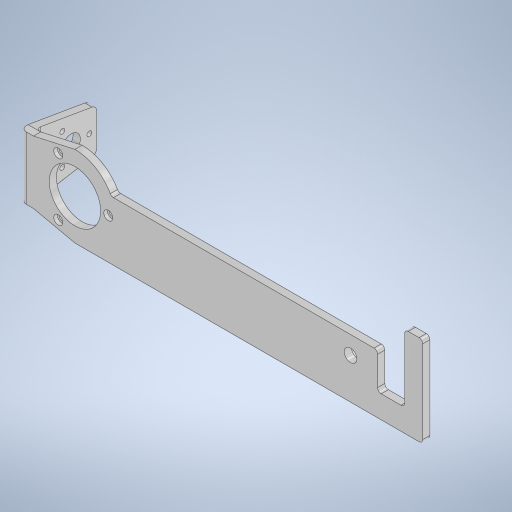
# Autodesk Inventor part: motor_holder_2
Saved by Autodesk Inventor 2024 (Build 280153000, 153)
## iProperties
Created: 2025-02-07
Part Number: motor_holder_2
Material: アルミニウム 6061
Document SubType Name: Modeling
Designer: 1412z
Density: 2.7 g/cm^3
Appearance: アルミニウム - つや出し
Author: 1412z
Autodesk Inventor part; units mm, degrees
ref_plane "YZ Plane" through (0, 0, 0) normal (1, 0, 0) x (0, 1, 0)
ref_plane "XZ Plane" through (0, 0, 0) normal (0, 1, 0) x (-1, 0, 0)
ref_plane "XY Plane" through (0, 0, 0) normal (0, 0, 1) x (1, 0, 0)
sketch "スケッチ1" plane through (0, 0, 0) normal (1, 0, 0) x (0, 1, 0)
  circle A0 centre (0, 0) radius 10
  circle A1 centre (0, -10) radius 1.35
  circle A2 centre (8.6603, 5) radius 1.35
  circle A3 centre (-8.6603, 5) radius 1.35
  circle A4 centre (0, 0) radius 5
  line L0 (0, 0) -> (0, 50)
  circle A5 centre (0, 50) radius 22.5
  circle A6 centre (0, 0) radius 14
  line L1 (-14, 0) -> (-22.5, 50)
  line L2 (14, 0) -> (22.5, 50)
  line L3 (0, -14) -> (-11.62, -14)
  line L4 (-11.62, -14) -> (-14, 0)
  line L5 (0, -14) -> (11.62, -14)
  line L6 (11.62, -14) -> (14, 0)
  line L7 (0, 20) -> (-17.4, 20)
  line L8 (0, 20) -> (17.4, 20)
  dimension "d0" = 20
  dimension "d1" = 2.7
  dimension "d4" = 360
  dimension "d6" = 10
  dimension "d7" = 50
  dimension "d8" = 45
  dimension "d9" = 28
  constraints: 18 end point, 7 point on line, 6 centre point, 6 coincident, 5 point on circle, 1 horizontal, 1 perpendicular, 1 tangent, 1 vertical, 1 vertical alignment, 10 other
  measures "d1" diameter of A1
  measures "d6" diameter of A4
  measures "d7" distance of L0.start L0.end
  measures "d8" diameter of A5
  measures "d9" diameter of A6
extrude "押し出し1" add sketch "スケッチ1" along normal blind 4 contours A0 A1 A3 A2 | A6 L6 L4 | A6 L1 L7 L0 | L0 L8 L2 A6 | L6 L5 A6 | A6 L3 L4
sketch "スケッチ2" plane through (0, -17.4, 20) normal (0, 0, 1) x (1, 0, 0)
  line L0 (0, 17.4) -> (30, 17.4)
  circle A0 centre (30, 17.4) radius 22.5
  circle A1 centre (30, 17.4) radius 18.5
  circle A2 centre (30, 17.4) radius 14.25
  circle A3 centre (48.5, 17.4) radius 1.35
  circle A4 centre (20.75, 33.4215) radius 1.35
  circle A5 centre (20.75, 1.3785) radius 1.35
  line L1 (0, 29.02) -> (0, 34.8) projected
  line L2 (0, 0) -> (0, 5.78) projected
  line L3 (0, 34.8) -> (0, 0)
  line L4 (4, 29.02) -> (4, 34.8) projected
  line L5 (4, 34.8) -> (7, 34.8)
  line L6 (7, 34.8) -> (30, 39.9)
  line L7 (4, 0) -> (4, 5.78) projected
  line L8 (4, 0) -> (7, 0)
  line L9 (7, 0) -> (30, -5.1)
  line L10 (4, 0) -> (0, 0)
  line L11 (0, 34.8) -> (4, 34.8) projected
  line L12 (0, 0) -> (0, 34.8)
  line L13 (0, 34.8) -> (4, 34.8)
  dimension "d14" = 37
  dimension "d12" = 30
  dimension "d13" = 45
  dimension "d15" = 28.5
  dimension "d16" = 2.7
  dimension "d19" = 360
  dimension "d21" = 3
  dimension "d22" = 3
  constraints: 18 end point, 5 centre point, 4 horizontal, 3 coincident, 2 point on circle, 1 collinear, 1 horizontal alignment, 1 perpendicular, 1 vertical, 9 other
  measures "d12" distance of L0.start L0.end
  measures "d13" diameter of A0
  measures "d15" diameter of A2
  measures "d16" diameter of A3
  measures "d21" distance of L4.end L5.end
  measures "d22" distance of L7.start L8.end
extrude "押し出し2" add sketch "スケッチ2" along normal blind 4 contours L3 L1 L11 L5 L6 A0 L0 | L0 A0 L9 L8 L10 L2 L3 | A1 A4 A3 A5 | A0 L6 L9
fillet "フィレット1" radius 3 2 edges at (4, 0, 20) (0, 0, 24)
fillet "フィレット2" radius 3 2 edges at (2, -11.62, -14) (2, 11.62, -14)
sketch "スケッチ7" plane through (0, -17.4, 24) normal (0, 0, 1) x (1, 0, 0)
  circle A0 centre (30, 17.4) radius 14.25 projected
  line L0 (30, 17.4) -> (182.95, 17.4)
  line L1 (30, 17.4) -> (182.95, 17.4) construction
  circle A1 centre (182.95, 17.4) radius 3.5
  circle A2 centre (182.95, 17.4) radius 10
  line L2 (182.95, 27.4) -> (50.1556, 27.4)
  arc A3 (30, -5.1) -> (30, 39.9) centre (30, 17.4) ccw projected
  line L3 (182.95, 27.4) -> (315.7444, 27.4) construction
  line L4 (182.95, 7.4) -> (50.1556, 7.4)
  point P0 (0, 17.4)
  dimension "d55" = 152.95
  dimension "d56" = 0
  dimension "d57" = 7
  dimension "d58" = 20
  dimension "d59" = 180
  constraints: 10 end point, 4 horizontal, 4 point on circle, 2 centre point, 2 coincident, 2 collinear, 1 tangent
  measures "d55" distance of L0.start L0.end
  measures "d56" distance between parallel lines of L0 L1
  measures "d57" diameter of A1
  measures "d58" diameter of A2
  measures "d59" angle of L2 L3
extrude "押し出し7" add sketch "スケッチ7" against normal blind 4 contours A3 L2 A2 L0 | L0 A2 L4 A3 | A2
sketch "スケッチ8" plane through (0, -17.4, 24) normal (0, 0, 1) x (1, 0, 0)
  circle A0 centre (20.75, 33.4215) radius 1.35 projected
  circle A1 centre (20.75, 33.4215) radius 2.5
  circle A2 centre (48.5, 17.4) radius 1.35 projected
  circle A3 centre (48.5, 17.4) radius 2.5
  circle A4 centre (20.75, 1.3785) radius 1.35 projected
  circle A5 centre (20.75, 1.3785) radius 2.5
  point P0 (0, 17.4)
  dimension "d63" = 5
  dimension "d64" = 5
  dimension "d65" = 5
  constraints: 3 centre point, 3 coincident
  measures "d63" diameter of A1
  measures "d64" diameter of A3
  measures "d65" diameter of A5
extrude "押し出し8" cut sketch "スケッチ8" against normal blind 2 contours A0 | A1 | A3 | A4 | A5
sketch "スケッチ9" plane through (0, -17.4, 24) normal (0, 0, 1) x (1, 0, 0)
  line L0 (50.1556, 27.4) -> (182.95, 27.4) projected
  line L1 (182.95, 27.4) -> (197.95, 27.4)
  line L2 (7, 0) -> (30, -5.1) projected
  line L3 (30, -5.1) -> (197.95, -5.1)
  line L4 (197.95, -5.1) -> (197.95, 27.4)
  line L5 (197.95, -5.1) -> (222.95, -5.1)
  line L6 (222.95, -5.1) -> (222.95, 44.9)
  line L7 (222.95, 44.9) -> (212.95, 44.9)
  line L8 (197.95, 7.4) -> (212.95, 7.4)
  line L9 (212.95, 7.4) -> (212.95, 44.9)
  circle A0 centre (182.95, 17.4) radius 3.5 projected
  circle A1 centre (182.95, 17.4) radius 10
  circle A2 centre (30, 17.4) radius 14.25 projected
  circle A3 centre (30, 17.4) radius 22.5
  line L10 (182.95, 7.4) -> (50.1556, 7.4) projected
  line L11 (50.1556, 7.4) -> (182.95, 7.4)
  point P0 (0, 17.4)
  point P1 (192.95, 17.4)
  point P2 (20.4894, -2.9911)
  dimension "d68" = 15
  dimension "d69" = 25
  dimension "d70" = 50
  dimension "d71" = 10
  constraints: 18 end point, 4 perpendicular, 3 horizontal, 2 coincident, 2 point on line, 1 centre point, 1 collinear, 1 point on circle, 2 other
  measures "d68" distance of L0.end L1.end
  measures "d69" distance of L3.end L5.end
  measures "d70" distance of L5.end L6.end
  measures "d71" distance of L6.end L7.end
extrude "押し出し9" add sketch "スケッチ9" against normal blind 4 contours L0 A1 L10 A3 | L1 L4 L3 A3 L10 A1 | L8 L9 L7 L6 L5 L4
fillet "フィレット4" radius 2 7 edges at (197.95, 10, 22) (50.1556, 10, 22) (212.95, 27.5, 22) (212.95, -10, 22) (222.95, 27.5, 22) (197.95, -10, 22) (222.95, -22.5, 22)
